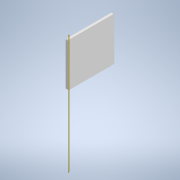
# Autodesk Inventor part: cover_wires
Saved by Autodesk Inventor 2020 (Build 240168000, 168)
## iProperties
Created: 2020-01-09
Part Number: cover_wires
Material: Generic
Document SubType Name: Modeling
Designer: erwin
Density: 1 g/cm^3
Appearance: Default
Author: erwin
Autodesk Inventor part; units mm, degrees
ref_plane "YZ Plane" through (0, 0, 0) normal (1, 0, 0) x (0, 1, 0)
ref_plane "XZ Plane" through (0, 0, 0) normal (0, 1, 0) x (-1, 0, 0)
ref_plane "XY Plane" through (0, 0, 0) normal (0, 0, 1) x (1, 0, 0)
ref_plane "Work Plane1" through (2, 85, 71.8) normal (-1, 0, 0) x (0, -1, 0)
sketch "Sketch1" plane through (2, 85, 71.8) normal (-1, 0, 0) x (0, -1, 0)
  line L0 (66.8, 0.8) -> (66.8, -70.8) projected
  line L1 (-1.8, 1.8) -> (66.8, 1.8)
  line L2 (66.8, 1.8) -> (66.8, -70.8)
  line L3 (66.8, -70.8) -> (-1.8, -70.8)
  line L4 (-1.8, -70.8) -> (-1.8, 1.8)
  point P0 (85, -71.8)
  point P1 (66.8, 1.8)
  point P2 (66.8, 0.8)
  constraints: 8 end point, 2 parallel, 1 horizontal, 1 perpendicular, 1 other
extrude "Extrusion1" add sketch "Sketch1" along normal blind 3.6
chamfer "Chamfer1" distance 1 angle 45 4 edges at (0.2, 86.8, 73.6) (0.2, 18.2, 73.6) (0.2, 86.8, 1) (0.2, 18.2, 1)
equation "\"d0\" = wood_thickness"
equation "\"wood_thickness\" = 3.6"
body "Solid1"
